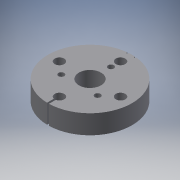
# Autodesk Inventor part: проставка
Saved by Autodesk Inventor 2019 (Build 230136000, 136)
## iProperties
Created: 2019-08-05
Part Number: проставка
Material: Типовые
Document SubType Name: Modeling
Designer: Петров Иван
Density: 1 g/cm^3
Appearance: По умолчанию
Author: Петров Иван
Autodesk Inventor part; units mm, degrees
ref_plane "YZ Plane" through (0, 0, 0) normal (1, 0, 0) x (0, 1, 0)
ref_plane "XZ Plane" through (0, 0, 0) normal (0, 1, 0) x (-1, 0, 0)
ref_plane "XY Plane" through (0, 0, 0) normal (0, 0, 1) x (1, 0, 0)
sketch "Эскиз1" plane through (0, 0, 0) normal (0, 1, 0) x (-1, 0, 0)
  arc A0 (-0.25, 9.2247) -> (0.25, 9.2247) centre (0, 8) ccw
  line L0 (-0.25, 10.9972) -> (-0.25, 9.2247)
  arc A1 (-0.25, 10.9972) -> (-1.1469, -10.94) centre (0, 0) ccw
  line L1 (-1.1469, -10.6297) -> (-1.1469, -10.94)
  line L2 (-0.8473, -10.6297) -> (-1.1469, -10.6297)
  line L3 (-0.8473, -10.9673) -> (-0.8473, -10.6297)
  arc A2 (-0.8473, -10.9673) -> (0.8535, -10.9668) centre (0, 0) ccw
  line L4 (0.8535, -10.6297) -> (0.8535, -10.9668)
  line L5 (1.1541, -10.6297) -> (0.8535, -10.6297)
  line L6 (1.1541, -10.9393) -> (1.1541, -10.6297)
  arc A3 (1.1541, -10.9393) -> (0.25, 10.9972) centre (0, 0) ccw
  line L7 (0.25, 9.2247) -> (0.25, 10.9972)
  circle A4 centre (8, 0) radius 1.25
  circle A5 centre (0, -8) radius 1.25
  circle A6 centre (-8, 0) radius 1.25
  circle A7 centre (0, -5.5) radius 0.75
  circle A8 centre (4.7631, 2.75) radius 0.75
  circle A9 centre (-4.7631, 2.75) radius 0.75
  circle A10 centre (0, 0) radius 2.9
  arc A11 (0.25, 9.2247) -> (-0.25, 9.2247) centre (0, 8) ccw
  constraints: 16 end point, 12 centre point, 10 point on circle
extrude "Выдавливание1" add sketch "Эскиз1" along normal blind 5 contours A0 L7 A3 L6 L5 L4 A2 L3 L2 L1 A1 L0
